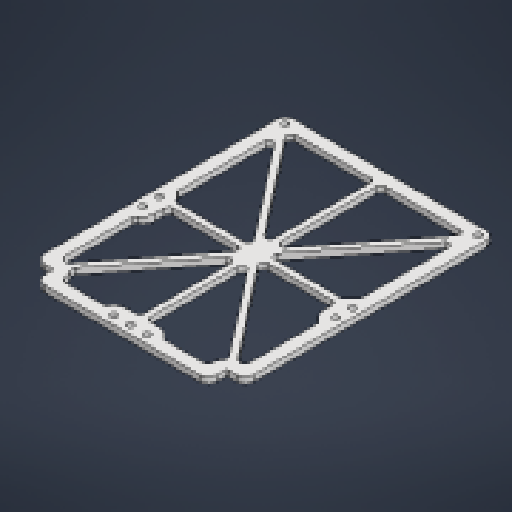
# Autodesk Inventor part: PLATE,KICKER,BACK
Saved by Autodesk Inventor 2026 (Build 300175000, 175)
## iProperties
Created: 2026-02-08
Part Number: PLATE,KICKER,BACK
Material: Generic
Document SubType Name: Sheet Metal
Designer: Owen L
Mass: 50.5573 g
Surface Area: 341.636 cm^2
Volume: 50.5573 cm^3
Density: 1 g/cm^3
Sheet Metal Rule: Default
Appearance: Default
Author: Owen L
Autodesk Inventor part; units mm, degrees
ref_plane "YZ Plane" through (0, 0, 0) normal (1, 0, 0) x (0, 1, 0)
ref_plane "XZ Plane" through (0, 0, 0) normal (0, 1, 0) x (-1, 0, 0)
ref_plane "XY Plane" through (0, 0, 0) normal (0, 0, 1) x (1, 0, 0)
sketch "Sketch1" plane through (0, 0, 0) normal (0, 1, 0) x (-1, 0, 0)
  line L0 (-79.375, 101.6) -> (79.375, 101.6)
  line L1 (79.375, 101.6) -> (79.375, -101.6)
  line L2 (79.375, -101.6) -> (-79.375, -101.6)
  line L3 (-79.375, -101.6) -> (-79.375, 101.6)
  line L4 (-79.375, 101.6) -> (79.375, -101.6) construction
  line L5 (79.375, 101.6) -> (-79.375, -101.6) construction
  line L6 (-79.375, 101.6) -> (-65.405, 101.6)
  line L7 (-65.405, 101.6) -> (-65.405, 87.63)
  line L8 (-65.405, 87.63) -> (-79.375, 87.63)
  line L9 (-79.375, 87.63) -> (-79.375, 101.6)
  line L10 (79.375, 101.6) -> (65.405, 101.6)
  line L11 (65.405, 101.6) -> (65.405, 87.63)
  line L12 (65.405, 87.63) -> (79.375, 87.63)
  line L13 (79.375, 87.63) -> (79.375, 101.6)
  point P0 (0, 0)
  dimension "d0" = 158.75
  dimension "d1" = 203.2
  dimension "d3" = 13.97
  measures "d0" distance of L1.end L2.end
  measures "d1" distance of L0.end L1.end
  measures "d3" distance of L6.end L7.end
extrude "Plate1" add sketch "Sketch1" along normal blind 4.7625 contours L0 L11 L12 L1 L2 L3 L8 L7
fillet "Corner Round1" radius 6.35 6 edges at (79.375, 2.3813, 87.63) (65.405, 2.3813, 101.6) (-79.375, 2.3813, 87.63) (-65.405, 2.3813, 101.6) (-79.375, 2.3813, -101.6) (79.375, 2.3813, -101.6)
fillet "Corner Round1" radius 1.143 2 edges at (65.405, 2.3813, 87.63) (-65.405, 2.3813, 87.63)
sketch "Sketch2" plane through (0, 4.7625, 0) normal (0, 1, 0) x (1, 0, 0)
  line L0 (79.375, 95.25) -> (79.375, -81.28) projected
  line L1 (-79.375, -81.28) -> (-79.375, 95.25) projected
  line L2 (59.055, -101.6) -> (-59.055, -101.6) projected
  line L3 (-73.025, 101.6) -> (73.025, 101.6) projected
  point P0 (0, 0)
  point P1 (73.025, -12.7)
  point P2 (73.025, 0)
  point P3 (-73.025, -12.7)
  point P4 (-73.025, 0)
  point P5 (0, -95.25)
  point P6 (12.7, -95.25)
  point P7 (-12.7, -95.25)
  point P8 (0, 101.6)
  point P9 (73.025, 95.25)
  point P10 (-73.025, 95.25)
  dimension "d7" = 12.7
  dimension "d8" = 6.35
  dimension "d10" = 6.35
  dimension "d18" = 12.7
  dimension "d19" = 12.7
  dimension "d20" = 6.35
  dimension "d31" = 6.35
  constraints: 6 horizontal alignment, 5 vertical alignment, 1 midpoint
  measures "d7" distance of point (73.025, -12.7) point (73.025, 0)
  measures "d8" distance from line of L0 point (73.025, 0)
  measures "d10" distance from line of L1 point (-73.025, 0)
  measures "d18" distance of point (0, -95.25) point (12.7, -95.25)
  measures "d19" distance of point (-12.7, -95.25) point (0, -95.25)
  measures "d20" distance from line of L2 point (0, -95.25)
  measures "d31" distance from line of L3 point (-73.025, 95.25)
hole "Hole1" at (-12.7, 4.7625, 95.25) at (12.7, 4.7625, 95.25) at (0, 4.7625, 95.25) at (-73.025, 4.7625, 0) at (-73.025, 4.7625, 12.7) at (73.025, 4.7625, 0) at (73.025, 4.7625, 12.7) at (73.025, 4.7625, -95.25) at (-73.025, 4.7625, -95.25) direction (0, -1, 0) diameter 4.9784 depth 4.7625 tip angle 118 clearance for "Flat Head Machine Screw (82)" size "#10" standard "Ansi Unified Screw Threads"
sketch "Sketch3" plane through (0, 4.7625, 0) normal (0, 1, 0) x (1, 0, 0)
  circle A0 centre (73.025, -12.7) radius 2.4892 projected
  circle A1 centre (73.025, 0) radius 2.4892 projected
  circle A2 centre (-73.025, -12.7) radius 2.4892 projected
  circle A3 centre (-73.025, 0) radius 2.4892 projected
  circle A4 centre (0, -95.25) radius 2.4892 projected
  circle A5 centre (12.7, -95.25) radius 2.4892 projected
  circle A6 centre (-12.7, -95.25) radius 2.4892 projected
  arc A7 (79.375, 95.25) -> (73.025, 101.6) centre (73.025, 95.25) ccw projected
  line L0 (-73.025, 101.6) -> (73.025, 101.6) projected
  arc A8 (-73.025, 101.6) -> (-79.375, 95.25) centre (-73.025, 95.25) ccw projected
  line L1 (-79.375, -81.28) -> (-79.375, 95.25) projected
  arc A9 (-79.375, -81.28) -> (-73.025, -87.63) centre (-73.025, -81.28) ccw projected
  line L2 (-66.548, -87.63) -> (-73.025, -87.63) projected
  arc A10 (-65.405, -88.773) -> (-66.548, -87.63) centre (-66.548, -88.773) ccw projected
  line L3 (-65.405, -95.25) -> (-65.405, -88.773) projected
  arc A11 (-65.405, -95.25) -> (-59.055, -101.6) centre (-59.055, -95.25) ccw projected
  line L4 (59.055, -101.6) -> (-59.055, -101.6) projected
  arc A12 (59.055, -101.6) -> (65.405, -95.25) centre (59.055, -95.25) ccw projected
  line L5 (65.405, -88.773) -> (65.405, -95.25) projected
  arc A13 (66.548, -87.63) -> (65.405, -88.773) centre (66.548, -88.773) ccw projected
  line L6 (73.025, -87.63) -> (66.548, -87.63) projected
  arc A14 (73.025, -87.63) -> (79.375, -81.28) centre (73.025, -81.28) ccw projected
  line L7 (79.375, 95.25) -> (79.375, -81.28) projected
  line L8 (-55.88, -92.075) -> (-55.88, -88.773)
  arc A15 (-55.88, -88.773) -> (-66.548, -78.105) centre (-66.548, -88.773) ccw
  line L9 (-66.548, -78.105) -> (-69.85, -78.105)
  line L10 (-69.85, -78.105) -> (-69.85, 92.075)
  line L11 (-69.85, 92.075) -> (69.85, 92.075)
  line L12 (69.85, 92.075) -> (69.85, -78.105)
  line L13 (69.85, -78.105) -> (66.548, -78.105)
  arc A16 (66.548, -78.105) -> (55.88, -88.773) centre (66.548, -88.773) ccw
  line L14 (55.88, -88.773) -> (55.88, -92.075)
  line L15 (55.88, -92.075) -> (-55.88, -92.075)
  arc A17 (21.6803, -92.075) -> (12.7, -85.725) centre (12.7, -95.25) ccw
  arc A18 (-12.7, -85.725) -> (-21.6803, -92.075) centre (-12.7, -95.25) ccw
  arc A19 (-69.85, -21.6803) -> (-63.5, -12.7) centre (-73.025, -12.7) ccw
  arc A20 (-63.5, 0) -> (-69.85, 8.9803) centre (-73.025, 0) ccw
  arc A21 (63.5, -12.7) -> (69.85, -21.6803) centre (73.025, -12.7) ccw
  arc A22 (69.85, 8.9803) -> (63.5, 0) centre (73.025, 0) ccw
  line L16 (12.7, -85.725) -> (-12.7, -85.725)
  line L17 (63.5, -12.7) -> (63.5, 0)
  line L18 (-63.5, 0) -> (-63.5, -12.7)
  line L19 (79.375, -101.6) -> (-79.375, 101.6) construction
  line L20 (81.2515, -100.134) -> (-77.4985, 103.066)
  line L21 (-81.2515, 100.134) -> (77.4985, -103.066)
  arc A23 (77.4985, -103.066) -> (81.2515, -100.134) centre (79.375, -101.6) ccw
  arc A24 (-77.4985, 103.066) -> (-81.2515, 100.134) centre (-79.375, 101.6) ccw
  line L22 (79.375, 101.6) -> (-79.375, -101.6) construction
  line L23 (77.4985, 103.066) -> (-81.2515, -100.134)
  line L24 (-77.4985, -103.066) -> (81.2515, 100.134)
  arc A25 (81.2515, 100.134) -> (77.4985, 103.066) centre (79.375, 101.6) ccw
  arc A26 (-81.2515, -100.134) -> (-77.4985, -103.066) centre (-79.375, -101.6) ccw
  line L25 (73.025, 0) -> (-73.025, 0) construction
  line L26 (73.025, 2.4892) -> (-73.025, 2.4892)
  line L27 (-73.025, -2.4892) -> (73.025, -2.4892)
  arc A27 (73.025, -2.4892) -> (73.025, 2.4892) centre (73.025, 0) ccw
  arc A28 (-73.025, 2.4892) -> (-73.025, -2.4892) centre (-73.025, 0) ccw
  line L28 (0, -95.25) -> (0, 95.25) construction
  line L29 (2.3813, -95.25) -> (2.3812, 95.25)
  line L30 (-2.3812, 95.25) -> (-2.3813, -95.25)
  arc A29 (-2.3813, -95.25) -> (2.3813, -95.25) centre (0, -95.25) ccw
  arc A30 (2.3812, 95.25) -> (-2.3812, 95.25) centre (0, 95.25) ccw
  point P0 (0, 0)
  point P1 (-21.6803, 92.075)
  point P2 (21.6803, 92.075)
  point P3 (0, 0)
  point P4 (0, 0)
  point P5 (0, 0)
  point P6 (0, 0)
  point P7 (-63.831, 2.4892)
  point P8 (-4.9665, 2.4892)
  point P9 (-69.85, 85.5401)
  point P10 (4.9665, 2.4892)
  point P11 (63.831, 2.4892)
  point P12 (69.85, 85.5401)
  point P13 (2.3813, 6.9159)
  point P14 (68.9118, 92.075)
  point P15 (-2.3813, 6.9159)
  point P16 (-68.9118, 92.075)
  point P17 (-64.2389, -78.3579)
  point P18 (-4.9665, -2.4892)
  point P19 (-63.5, -2.4892)
  point P20 (-2.3813, -85.725)
  point P21 (-2.3813, -6.9159)
  point P22 (-59.8471, -80.4722)
  point P23 (63.5, -2.4892)
  point P24 (4.9665, -2.4892)
  point P25 (64.2389, -78.3579)
  point P26 (59.8471, -80.4722)
  point P27 (2.3813, -6.9159)
  point P28 (2.3813, -85.725)
  point P29 (2.3813, -0.8199)
  point P30 (2.3813, -92.075)
  point P31 (-2.3813, 0.8199)
  point P32 (-2.3813, 92.075)
  point P33 (-2.3813, -92.075)
  point P34 (2.3813, 92.075)
  point P35 (2.3813, 0.8199)
  point P36 (-2.3813, -0.8199)
  dimension "d22" = 9.525
  dimension "d23" = 9.525
  dimension "d24" = 4.7625
  dimension "d25" = 4.7625
  dimension "d26" = 4.9784
  dimension "d27" = 4.7625
  constraints: 54 end point, 32 point on circle, 22 tangent, 16 centre point, 16 point on line, 6 coincident, 6 equal radius, 4 midpoint, 4 parallel, 2 perpendicular, 9 other
  measures "d22" distance between parallel lines of L4 L15
  measures "d23" radius of A17
  measures "d24" diameter of A24
  measures "d25" diameter of A26
  measures "d26" diameter of A28
  measures "d27" diameter of A30
extrude "Cut1" cut sketch "Sketch3" against normal blind 4.7625 contours A22 L26 L24 L12 | L12 L13 A16 L20 L27 L17 A21 | L23 L29 L11 | A16 L14 L15 A17 L16 L29 L21 | L30 L20 L11 | L30 L16 A18 L15 L8 A15 L24 | L26 A20 L10 L21 | L23 A15 L9 L10 A19 L18 L27
fillet "Corner Round2" radius 3.175 34 edges at (4.9665, 2.3813, 2.4892) (2.3813, 2.3813, -6.9159) (-63.5, 2.3813, 2.4892) (69.85, 2.3813, 21.6803) (63.5, 2.3813, 2.4892) (-69.85, 2.3813, -85.5401) (-69.85, 2.3813, -8.9803) (-4.9665, 2.3813, -2.4892) (-68.9118, 2.3813, -92.075) (-69.85, 2.3813, 21.6803) (-63.831, 2.3813, -2.4892) (55.88, 2.3813, 92.075) (21.6803, 2.3813, 92.075) (2.3813, 2.3813, 85.725) (2.3813, 2.3813, 6.9159) (-4.9665, 2.3813, 2.4892) (-69.85, 2.3813, 78.105) (-2.3813, 2.3813, 6.9159) (-2.3813, 2.3813, 85.725) (-21.6803, 2.3813, 92.075) (-59.8471, 2.3813, 80.4722) (-64.2389, 2.3813, 78.3579) (68.9118, 2.3813, -92.075) (-2.3813, 2.3813, -6.9159) (4.9665, 2.3813, -2.4892) (63.831, 2.3813, -2.4892) (69.85, 2.3813, -8.9803) (69.85, 2.3813, -85.5401) (-55.88, 2.3813, 92.075) (69.85, 2.3813, 78.105) (59.8471, 2.3813, 80.4722) (64.2389, 2.3813, 78.3579) (-2.3813, 2.3813, -92.075) (2.3813, 2.3813, -92.075)
equation "\"d16\" = Thickness"
equation "\"d28\" = Thickness"
equation "\"d4\" = Thickness"
equation "\"BendRadius\" = Thickness"
equation "\"BendReliefWidth\" = Thickness"
equation "\"BendReliefDepth\" = 0.5 * Thickness"
equation "\"CornerReliefSize\" = 4 * Thickness"
equation "\"MinimumRemnant\" = 2 * Thickness"
equation "\"TransitionRadius\" = BendRadius"
equation "\"JacobiRadiusSize\" = BendRadius"
equation "\"GapSize\" = Thickness"
equation "\"Thickness\" = 4.7625"
body "Solid1"
